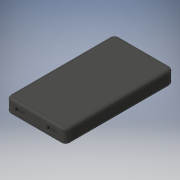
# Autodesk Inventor part: Battery
Saved by Autodesk Inventor 2016 (Build 200138000, 138)
## iProperties
Created: 2016-05-23
Part Number: Battery
Material: Generic
Document SubType Name: Modeling
Designer: kromm.je.s
Density: 1 g/cm^3
Appearance: Rubber - Black
Author: kromm.je.s
Autodesk Inventor part; units mm, degrees
ref_plane "YZ Plane" through (0, 0, 0) normal (1, 0, 0) x (0, 1, 0)
ref_plane "XZ Plane" through (0, 0, 0) normal (0, 1, 0) x (-1, 0, 0)
ref_plane "XY Plane" through (0, 0, 0) normal (0, 0, 1) x (1, 0, 0)
sketch "Sketch1" plane through (0, 0, 0) normal (0, 1, 0) x (-1, 0, 0)
  line L0 (0, 0) -> (82.042, 0)
  line L1 (82.042, 0) -> (82.042, -149.606)
  line L2 (82.042, -149.606) -> (0, -149.606)
  line L3 (0, -149.606) -> (0, 0)
  dimension "d0" = 82.042
  dimension "d1" = 149.606
  constraints: 8 end point, 2 parallel, 1 horizontal, 1 perpendicular
  measures "d0" distance of L1.end L2.end
  measures "d1" distance of L0.end L1.end
extrude "Extrusion1" add sketch "Sketch1" along normal blind 19.558
fillet "Fillet1" radius 6.35 4 edges at (0, 9.779, 0) (-82.042, 9.779, 0) (-82.042, 9.779, -149.606) (0, 9.779, -149.606)
fillet "Fillet2" radius 3.175 16 edges at (-80.1821, 19.558, -147.7461) (-82.042, 19.558, -74.803) (-80.1821, 19.558, -1.8599) (-41.021, 19.558, 0) (-1.8599, 19.558, -1.8599) (0, 19.558, -74.803) (-1.8599, 19.558, -147.7461) (-41.021, 19.558, -149.606) (-1.8599, 0, -1.8599) (-41.021, 0, 0) (-80.1821, 0, -1.8599) (-82.042, 0, -74.803) (-80.1821, 0, -147.7461) (-41.021, 0, -149.606) (-1.8599, 0, -147.7461) (0, 0, -74.803)
sketch "Sketch2" plane through (-75.692, 3.175, 0) normal (0, 0, 1) x (1, 0, 0)
  line L0 (69.342, 0) -> (0, 0) projected
  line L1 (69.342, 13.208) -> (69.342, 0) projected
  line L2 (0, 13.208) -> (69.342, 13.208) projected
  line L3 (0, 0) -> (0, 13.208) projected
  line L4 (0, 13.208) -> (0, 0) projected
  line L5 (0, 6.604) -> (12.7, 6.604)
  line L6 (69.342, 0) -> (69.342, 13.208) projected
  line L7 (69.342, 6.604) -> (56.642, 6.604)
  line L8 (6.35, 4.064) -> (19.05, 4.064)
  line L9 (19.05, 4.064) -> (19.05, 9.144)
  line L10 (19.05, 9.144) -> (6.35, 9.144)
  line L11 (6.35, 9.144) -> (6.35, 4.064)
  line L12 (6.35, 4.064) -> (19.05, 9.144) construction
  line L13 (19.05, 4.064) -> (6.35, 9.144) construction
  line L14 (50.292, 4.064) -> (62.992, 4.064)
  line L15 (62.992, 4.064) -> (62.992, 9.144)
  line L16 (62.992, 9.144) -> (50.292, 9.144)
  line L17 (50.292, 9.144) -> (50.292, 4.064)
  line L18 (50.292, 4.064) -> (62.992, 9.144) construction
  line L19 (62.992, 4.064) -> (50.292, 9.144) construction
  point P0 (75.692, -3.175)
  dimension "d6" = 12.7
  dimension "d7" = 12.7
  dimension "d8" = 12.7
  dimension "d9" = 5.08
  dimension "d10" = 12.7
  dimension "d11" = 5.08
  constraints: 28 end point, 6 midpoint, 4 parallel, 3 horizontal, 3 perpendicular
  measures "d6" distance of L5.start L5.end
  measures "d7" distance of L7.start L7.end
  measures "d8" distance of L10.end L9.end
  measures "d9" distance of L9.end L8.end
  measures "d10" distance of L16.end L15.end
  measures "d11" distance of L15.end L14.end
extrude "Extrusion2" cut sketch "Sketch2" against normal blind 3.175 contours L15 L14 L17 L16 | L11 L10 L9 L8
chamfer "Chamfer1" distance 0.7937 angle 45 8 edges at (-69.342, 9.779, 0) (-62.992, 12.319, 0) (-62.992, 7.239, 0) (-56.642, 9.779, 0) (-25.4, 9.779, 0) (-19.05, 12.319, 0) (-19.05, 7.239, 0) (-12.7, 9.779, 0)
body "Solid1"
